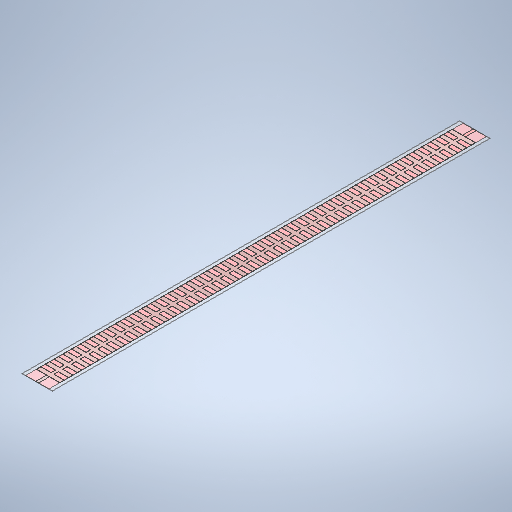
# Autodesk Inventor part: Sensor_completo
Saved by Autodesk Inventor 2025.2 (Build 292293000, 293)
## iProperties
Created: 2025-04-22
Part Number: Sensor_completo
Material: Genérico
Document SubType Name: Modeling
Designer: julia
Density: 1 g/cm^3
Appearance: Transparente - Claro
Author: julia
Autodesk Inventor part; units mm, degrees
ref_plane "YZ Plane" through (0, 0, 0) normal (1, 0, 0) x (0, 1, 0)
ref_plane "XZ Plane" through (0, 0, 0) normal (0, 1, 0) x (-1, 0, 0)
ref_plane "XY Plane" through (0, 0, 0) normal (0, 0, 1) x (1, 0, 0)
sketch "Boceto1" plane through (0, 0, 0) normal (0, 1, 0) x (-1, 0, 0)
  line L0 (0, 0) -> (1.034, 0)
  line L1 (1.026, -15) -> (0, -15)
  line L2 (0, -15) -> (0, 0)
  line L3 (1.034, 0) -> (0.517, 0)
  line L4 (0.517, 0) -> (0.6595, 0)
  line L5 (0.517, 0) -> (0.567, 0)
  line L6 (0.567, 0) -> (0.567, -0.375)
  line L7 (0.567, -0.375) -> (0.917, -0.375)
  line L8 (0.917, -0.375) -> (0.917, -0.525)
  line L9 (0.517, 0) -> (0.467, 0)
  line L10 (0.467, 0) -> (0.467, -0.375)
  line L11 (0.467, -0.375) -> (0.117, -0.375)
  line L12 (0.117, -0.375) -> (0.117, -0.525)
  line L13 (0.117, -0.525) -> (0.467, -0.525)
  line L14 (0.467, -0.525) -> (0.467, -0.675)
  line L15 (0.917, -0.525) -> (0.567, -0.525)
  line L16 (0.567, -0.525) -> (0.567, -0.675)
  line L17 (0.567, -14.625) -> (0.567, -15)
  line L18 (0.467, -14.625) -> (0.467, -15)
  line L19 (0.567, -14.625) -> (0.467, -14.625)
  line L20 (0.567, -0.375) -> (0.467, -0.375)
  line L21 (1.034, -15) -> (1.042, -15)
  line L22 (1.034, -15) -> (1.026, -15)
  line L23 (1.026, -15) -> (1.034, 0)
  line L24 (0.567, -0.675) -> (0.917, -0.675)
  line L25 (0.917, -0.675) -> (0.917, -0.825)
  line L26 (0.917, -0.825) -> (0.567, -0.825)
  line L27 (0.567, -0.825) -> (0.567, -0.975)
  line L28 (0.467, -0.675) -> (0.117, -0.675)
  line L29 (0.117, -0.675) -> (0.117, -0.825)
  line L30 (0.117, -0.825) -> (0.467, -0.825)
  line L31 (0.467, -0.825) -> (0.467, -0.975)
  line L32 (0.567, -0.975) -> (0.917, -0.975)
  line L33 (0.917, -0.975) -> (0.917, -1.125)
  line L34 (0.917, -1.125) -> (0.567, -1.125)
  line L35 (0.567, -1.125) -> (0.567, -1.275)
  line L36 (0.467, -0.975) -> (0.117, -0.975)
  line L37 (0.117, -0.975) -> (0.117, -1.125)
  line L38 (0.117, -1.125) -> (0.467, -1.125)
  line L39 (0.467, -1.125) -> (0.467, -1.275)
  line L40 (0.567, -1.275) -> (0.917, -1.275)
  line L41 (0.917, -1.275) -> (0.917, -1.425)
  line L42 (0.917, -1.425) -> (0.567, -1.425)
  line L43 (0.567, -1.425) -> (0.567, -1.575)
  line L44 (0.467, -1.275) -> (0.117, -1.275)
  line L45 (0.117, -1.275) -> (0.117, -1.425)
  line L46 (0.117, -1.425) -> (0.467, -1.425)
  line L47 (0.467, -1.425) -> (0.467, -1.575)
  line L48 (0.567, -1.575) -> (0.917, -1.575)
  line L49 (0.917, -1.575) -> (0.917, -1.725)
  line L50 (0.917, -1.725) -> (0.567, -1.725)
  line L51 (0.567, -1.725) -> (0.567, -1.875)
  line L52 (0.467, -1.575) -> (0.117, -1.575)
  line L53 (0.117, -1.575) -> (0.117, -1.725)
  line L54 (0.117, -1.725) -> (0.467, -1.725)
  line L55 (0.467, -1.725) -> (0.467, -1.875)
  line L56 (0.567, -1.875) -> (0.917, -1.875)
  line L57 (0.917, -1.875) -> (0.917, -2.025)
  line L58 (0.917, -2.025) -> (0.567, -2.025)
  line L59 (0.567, -2.025) -> (0.567, -2.175)
  line L60 (0.467, -1.875) -> (0.117, -1.875)
  line L61 (0.117, -1.875) -> (0.117, -2.025)
  line L62 (0.117, -2.025) -> (0.467, -2.025)
  line L63 (0.467, -2.025) -> (0.467, -2.175)
  line L64 (0.567, -2.175) -> (0.917, -2.175)
  line L65 (0.917, -2.175) -> (0.917, -2.325)
  line L66 (0.917, -2.325) -> (0.567, -2.325)
  line L67 (0.567, -2.325) -> (0.567, -2.475)
  line L68 (0.467, -2.175) -> (0.117, -2.175)
  line L69 (0.117, -2.175) -> (0.117, -2.325)
  line L70 (0.117, -2.325) -> (0.467, -2.325)
  line L71 (0.467, -2.325) -> (0.467, -2.475)
  line L72 (0.567, -2.475) -> (0.917, -2.475)
  line L73 (0.917, -2.475) -> (0.917, -2.625)
  line L74 (0.917, -2.625) -> (0.567, -2.625)
  line L75 (0.567, -2.625) -> (0.567, -2.775)
  line L76 (0.467, -2.475) -> (0.117, -2.475)
  line L77 (0.117, -2.475) -> (0.117, -2.625)
  line L78 (0.117, -2.625) -> (0.467, -2.625)
  line L79 (0.467, -2.625) -> (0.467, -2.775)
  line L80 (0.567, -2.775) -> (0.917, -2.775)
  line L81 (0.917, -2.775) -> (0.917, -2.925)
  line L82 (0.917, -2.925) -> (0.567, -2.925)
  line L83 (0.567, -2.925) -> (0.567, -3.075)
  line L84 (0.467, -2.775) -> (0.117, -2.775)
  line L85 (0.117, -2.775) -> (0.117, -2.925)
  line L86 (0.117, -2.925) -> (0.467, -2.925)
  line L87 (0.467, -2.925) -> (0.467, -3.075)
  line L88 (0.567, -3.075) -> (0.917, -3.075)
  line L89 (0.917, -3.075) -> (0.917, -3.225)
  line L90 (0.917, -3.225) -> (0.567, -3.225)
  line L91 (0.567, -3.225) -> (0.567, -3.375)
  line L92 (0.467, -3.075) -> (0.117, -3.075)
  line L93 (0.117, -3.075) -> (0.117, -3.225)
  line L94 (0.117, -3.225) -> (0.467, -3.225)
  line L95 (0.467, -3.225) -> (0.467, -3.375)
  line L96 (0.567, -3.375) -> (0.917, -3.375)
  line L97 (0.917, -3.375) -> (0.917, -3.525)
  line L98 (0.917, -3.525) -> (0.567, -3.525)
  line L99 (0.567, -3.525) -> (0.567, -3.675)
  line L100 (0.467, -3.375) -> (0.117, -3.375)
  line L101 (0.117, -3.375) -> (0.117, -3.525)
  line L102 (0.117, -3.525) -> (0.467, -3.525)
  line L103 (0.467, -3.525) -> (0.467, -3.675)
  line L104 (0.567, -3.675) -> (0.917, -3.675)
  line L105 (0.917, -3.675) -> (0.917, -3.825)
  line L106 (0.917, -3.825) -> (0.567, -3.825)
  line L107 (0.567, -3.825) -> (0.567, -3.975)
  line L108 (0.467, -3.675) -> (0.117, -3.675)
  line L109 (0.117, -3.675) -> (0.117, -3.825)
  line L110 (0.117, -3.825) -> (0.467, -3.825)
  line L111 (0.467, -3.825) -> (0.467, -3.975)
  line L112 (0.567, -3.975) -> (0.917, -3.975)
  line L113 (0.917, -3.975) -> (0.917, -4.125)
  line L114 (0.917, -4.125) -> (0.567, -4.125)
  line L115 (0.567, -4.125) -> (0.567, -4.275)
  line L116 (0.467, -3.975) -> (0.117, -3.975)
  line L117 (0.117, -3.975) -> (0.117, -4.125)
  line L118 (0.117, -4.125) -> (0.467, -4.125)
  line L119 (0.467, -4.125) -> (0.467, -4.275)
  line L120 (0.567, -4.275) -> (0.917, -4.275)
  line L121 (0.917, -4.275) -> (0.917, -4.425)
  line L122 (0.917, -4.425) -> (0.567, -4.425)
  line L123 (0.567, -4.425) -> (0.567, -4.575)
  line L124 (0.467, -4.275) -> (0.117, -4.275)
  line L125 (0.117, -4.275) -> (0.117, -4.425)
  line L126 (0.117, -4.425) -> (0.467, -4.425)
  line L127 (0.467, -4.425) -> (0.467, -4.575)
  line L128 (0.567, -4.575) -> (0.917, -4.575)
  line L129 (0.917, -4.575) -> (0.917, -4.725)
  line L130 (0.917, -4.725) -> (0.567, -4.725)
  line L131 (0.567, -4.725) -> (0.567, -4.875)
  line L132 (0.467, -4.575) -> (0.117, -4.575)
  line L133 (0.117, -4.575) -> (0.117, -4.725)
  line L134 (0.117, -4.725) -> (0.467, -4.725)
  line L135 (0.467, -4.725) -> (0.467, -4.875)
  line L136 (0.567, -4.875) -> (0.917, -4.875)
  line L137 (0.917, -4.875) -> (0.917, -5.025)
  line L138 (0.917, -5.025) -> (0.567, -5.025)
  line L139 (0.567, -5.025) -> (0.567, -5.175)
  line L140 (0.467, -4.875) -> (0.117, -4.875)
  line L141 (0.117, -4.875) -> (0.117, -5.025)
  line L142 (0.117, -5.025) -> (0.467, -5.025)
  line L143 (0.467, -5.025) -> (0.467, -5.175)
  line L144 (0.567, -5.175) -> (0.917, -5.175)
  line L145 (0.917, -5.175) -> (0.917, -5.325)
  line L146 (0.917, -5.325) -> (0.567, -5.325)
  line L147 (0.567, -5.325) -> (0.567, -5.475)
  line L148 (0.467, -5.175) -> (0.117, -5.175)
  line L149 (0.117, -5.175) -> (0.117, -5.325)
  line L150 (0.117, -5.325) -> (0.467, -5.325)
  line L151 (0.467, -5.325) -> (0.467, -5.475)
  line L152 (0.567, -5.475) -> (0.917, -5.475)
  line L153 (0.917, -5.475) -> (0.917, -5.625)
  line L154 (0.917, -5.625) -> (0.567, -5.625)
  line L155 (0.567, -5.625) -> (0.567, -5.775)
  line L156 (0.467, -5.475) -> (0.117, -5.475)
  line L157 (0.117, -5.475) -> (0.117, -5.625)
  line L158 (0.117, -5.625) -> (0.467, -5.625)
  line L159 (0.467, -5.625) -> (0.467, -5.775)
  line L160 (0.567, -5.775) -> (0.917, -5.775)
  line L161 (0.917, -5.775) -> (0.917, -5.925)
  line L162 (0.917, -5.925) -> (0.567, -5.925)
  line L163 (0.567, -5.925) -> (0.567, -6.075)
  line L164 (0.467, -5.775) -> (0.117, -5.775)
  line L165 (0.117, -5.775) -> (0.117, -5.925)
  line L166 (0.117, -5.925) -> (0.467, -5.925)
  line L167 (0.467, -5.925) -> (0.467, -6.075)
  line L168 (0.567, -6.075) -> (0.917, -6.075)
  line L169 (0.917, -6.075) -> (0.917, -6.225)
  line L170 (0.917, -6.225) -> (0.567, -6.225)
  line L171 (0.567, -6.225) -> (0.567, -6.375)
  line L172 (0.467, -6.075) -> (0.117, -6.075)
  line L173 (0.117, -6.075) -> (0.117, -6.225)
  line L174 (0.117, -6.225) -> (0.467, -6.225)
  line L175 (0.467, -6.225) -> (0.467, -6.375)
  line L176 (0.567, -6.375) -> (0.917, -6.375)
  line L177 (0.917, -6.375) -> (0.917, -6.525)
  line L178 (0.917, -6.525) -> (0.567, -6.525)
  line L179 (0.567, -6.525) -> (0.567, -6.675)
  line L180 (0.467, -6.375) -> (0.117, -6.375)
  line L181 (0.117, -6.375) -> (0.117, -6.525)
  line L182 (0.117, -6.525) -> (0.467, -6.525)
  line L183 (0.467, -6.525) -> (0.467, -6.675)
  line L184 (0.567, -6.675) -> (0.917, -6.675)
  line L185 (0.917, -6.675) -> (0.917, -6.825)
  line L186 (0.917, -6.825) -> (0.567, -6.825)
  line L187 (0.567, -6.825) -> (0.567, -6.975)
  line L188 (0.467, -6.675) -> (0.117, -6.675)
  line L189 (0.117, -6.675) -> (0.117, -6.825)
  line L190 (0.117, -6.825) -> (0.467, -6.825)
  line L191 (0.467, -6.825) -> (0.467, -6.975)
  line L192 (0.567, -6.975) -> (0.917, -6.975)
  line L193 (0.917, -6.975) -> (0.917, -7.125)
  line L194 (0.917, -7.125) -> (0.567, -7.125)
  line L195 (0.567, -7.125) -> (0.567, -7.275)
  line L196 (0.467, -6.975) -> (0.117, -6.975)
  line L197 (0.117, -6.975) -> (0.117, -7.125)
  line L198 (0.117, -7.125) -> (0.467, -7.125)
  line L199 (0.467, -7.125) -> (0.467, -7.275)
  line L200 (0.567, -7.275) -> (0.917, -7.275)
  line L201 (0.917, -7.275) -> (0.917, -7.425)
  line L202 (0.917, -7.425) -> (0.567, -7.425)
  line L203 (0.567, -7.425) -> (0.567, -7.575)
  line L204 (0.467, -7.275) -> (0.117, -7.275)
  line L205 (0.117, -7.275) -> (0.117, -7.425)
  line L206 (0.117, -7.425) -> (0.467, -7.425)
  line L207 (0.467, -7.425) -> (0.467, -7.575)
  line L208 (0.567, -7.575) -> (0.917, -7.575)
  line L209 (0.917, -7.575) -> (0.917, -7.725)
  line L210 (0.917, -7.725) -> (0.567, -7.725)
  line L211 (0.567, -7.725) -> (0.567, -7.875)
  line L212 (0.467, -7.575) -> (0.117, -7.575)
  line L213 (0.117, -7.575) -> (0.117, -7.725)
  line L214 (0.117, -7.725) -> (0.467, -7.725)
  line L215 (0.467, -7.725) -> (0.467, -7.875)
  line L216 (0.567, -7.875) -> (0.917, -7.875)
  line L217 (0.917, -7.875) -> (0.917, -8.025)
  line L218 (0.917, -8.025) -> (0.567, -8.025)
  line L219 (0.567, -8.025) -> (0.567, -8.175)
  line L220 (0.467, -7.875) -> (0.117, -7.875)
  line L221 (0.117, -7.875) -> (0.117, -8.025)
  line L222 (0.117, -8.025) -> (0.467, -8.025)
  line L223 (0.467, -8.025) -> (0.467, -8.175)
  line L224 (0.567, -8.175) -> (0.917, -8.175)
  line L225 (0.917, -8.175) -> (0.917, -8.325)
  line L226 (0.917, -8.325) -> (0.567, -8.325)
  line L227 (0.567, -8.325) -> (0.567, -8.475)
  line L228 (0.467, -8.175) -> (0.117, -8.175)
  line L229 (0.117, -8.175) -> (0.117, -8.325)
  line L230 (0.117, -8.325) -> (0.467, -8.325)
  line L231 (0.467, -8.325) -> (0.467, -8.475)
  line L232 (0.567, -8.475) -> (0.917, -8.475)
  line L233 (0.917, -8.475) -> (0.917, -8.625)
  line L234 (0.917, -8.625) -> (0.567, -8.625)
  line L235 (0.567, -8.625) -> (0.567, -8.775)
  line L236 (0.467, -8.475) -> (0.117, -8.475)
  line L237 (0.117, -8.475) -> (0.117, -8.625)
  line L238 (0.117, -8.625) -> (0.467, -8.625)
  line L239 (0.467, -8.625) -> (0.467, -8.775)
  line L240 (0.567, -8.775) -> (0.917, -8.775)
  line L241 (0.917, -8.775) -> (0.917, -8.925)
  line L242 (0.917, -8.925) -> (0.567, -8.925)
  line L243 (0.567, -8.925) -> (0.567, -9.075)
  line L244 (0.467, -8.775) -> (0.117, -8.775)
  line L245 (0.117, -8.775) -> (0.117, -8.925)
  line L246 (0.117, -8.925) -> (0.467, -8.925)
  line L247 (0.467, -8.925) -> (0.467, -9.075)
  line L248 (0.567, -9.075) -> (0.917, -9.075)
  line L249 (0.917, -9.075) -> (0.917, -9.225)
  line L250 (0.917, -9.225) -> (0.567, -9.225)
  line L251 (0.567, -9.225) -> (0.567, -9.375)
  line L252 (0.467, -9.075) -> (0.117, -9.075)
  line L253 (0.117, -9.075) -> (0.117, -9.225)
  line L254 (0.117, -9.225) -> (0.467, -9.225)
  line L255 (0.467, -9.225) -> (0.467, -9.375)
  line L256 (0.567, -9.375) -> (0.917, -9.375)
  line L257 (0.917, -9.375) -> (0.917, -9.525)
  line L258 (0.917, -9.525) -> (0.567, -9.525)
  line L259 (0.567, -9.525) -> (0.567, -9.675)
  line L260 (0.467, -9.375) -> (0.117, -9.375)
  line L261 (0.117, -9.375) -> (0.117, -9.525)
  line L262 (0.117, -9.525) -> (0.467, -9.525)
  line L263 (0.467, -9.525) -> (0.467, -9.675)
  line L264 (0.567, -9.675) -> (0.917, -9.675)
  line L265 (0.917, -9.675) -> (0.917, -9.825)
  line L266 (0.917, -9.825) -> (0.567, -9.825)
  line L267 (0.567, -9.825) -> (0.567, -9.975)
  line L268 (0.467, -9.675) -> (0.117, -9.675)
  line L269 (0.117, -9.675) -> (0.117, -9.825)
  line L270 (0.117, -9.825) -> (0.467, -9.825)
  line L271 (0.467, -9.825) -> (0.467, -9.975)
  line L272 (0.567, -9.975) -> (0.917, -9.975)
  line L273 (0.917, -9.975) -> (0.917, -10.125)
  line L274 (0.917, -10.125) -> (0.567, -10.125)
  line L275 (0.567, -10.125) -> (0.567, -10.275)
  line L276 (0.467, -9.975) -> (0.117, -9.975)
  line L277 (0.117, -9.975) -> (0.117, -10.125)
  line L278 (0.117, -10.125) -> (0.467, -10.125)
  line L279 (0.467, -10.125) -> (0.467, -10.275)
  line L280 (0.567, -10.275) -> (0.917, -10.275)
  line L281 (0.917, -10.275) -> (0.917, -10.425)
  line L282 (0.917, -10.425) -> (0.567, -10.425)
  line L283 (0.567, -10.425) -> (0.567, -10.575)
  line L284 (0.467, -10.275) -> (0.117, -10.275)
  line L285 (0.117, -10.275) -> (0.117, -10.425)
  line L286 (0.117, -10.425) -> (0.467, -10.425)
  line L287 (0.467, -10.425) -> (0.467, -10.575)
  line L288 (0.567, -10.575) -> (0.917, -10.575)
  line L289 (0.917, -10.575) -> (0.917, -10.725)
  line L290 (0.917, -10.725) -> (0.567, -10.725)
  line L291 (0.567, -10.725) -> (0.567, -10.875)
  line L292 (0.467, -10.575) -> (0.117, -10.575)
  line L293 (0.117, -10.575) -> (0.117, -10.725)
  line L294 (0.117, -10.725) -> (0.467, -10.725)
  line L295 (0.467, -10.725) -> (0.467, -10.875)
  line L296 (0.567, -10.875) -> (0.917, -10.875)
  line L297 (0.917, -10.875) -> (0.917, -11.025)
  line L298 (0.917, -11.025) -> (0.567, -11.025)
  line L299 (0.567, -11.025) -> (0.567, -11.175)
  line L300 (0.467, -10.875) -> (0.117, -10.875)
  line L301 (0.117, -10.875) -> (0.117, -11.025)
  line L302 (0.117, -11.025) -> (0.467, -11.025)
  line L303 (0.467, -11.025) -> (0.467, -11.175)
  line L304 (0.567, -11.175) -> (0.917, -11.175)
  line L305 (0.917, -11.175) -> (0.917, -11.325)
  line L306 (0.917, -11.325) -> (0.567, -11.325)
  line L307 (0.567, -11.325) -> (0.567, -11.475)
  line L308 (0.467, -11.175) -> (0.117, -11.175)
  line L309 (0.117, -11.175) -> (0.117, -11.325)
  line L310 (0.117, -11.325) -> (0.467, -11.325)
  line L311 (0.467, -11.325) -> (0.467, -11.475)
  line L312 (0.567, -11.475) -> (0.917, -11.475)
  line L313 (0.917, -11.475) -> (0.917, -11.625)
  line L314 (0.917, -11.625) -> (0.567, -11.625)
  line L315 (0.567, -11.625) -> (0.567, -11.775)
  line L316 (0.467, -11.475) -> (0.117, -11.475)
  line L317 (0.117, -11.475) -> (0.117, -11.625)
  line L318 (0.117, -11.625) -> (0.467, -11.625)
  line L319 (0.467, -11.625) -> (0.467, -11.775)
  line L320 (0.567, -11.775) -> (0.917, -11.775)
  line L321 (0.917, -11.775) -> (0.917, -11.925)
  line L322 (0.917, -11.925) -> (0.567, -11.925)
  line L323 (0.567, -11.925) -> (0.567, -12.075)
  line L324 (0.467, -11.775) -> (0.117, -11.775)
  line L325 (0.117, -11.775) -> (0.117, -11.925)
  line L326 (0.117, -11.925) -> (0.467, -11.925)
  line L327 (0.467, -11.925) -> (0.467, -12.075)
  line L328 (0.567, -12.075) -> (0.917, -12.075)
  line L329 (0.917, -12.075) -> (0.917, -12.225)
  line L330 (0.917, -12.225) -> (0.567, -12.225)
  line L331 (0.567, -12.225) -> (0.567, -12.375)
  line L332 (0.467, -12.075) -> (0.117, -12.075)
  line L333 (0.117, -12.075) -> (0.117, -12.225)
  line L334 (0.117, -12.225) -> (0.467, -12.225)
  line L335 (0.467, -12.225) -> (0.467, -12.375)
  line L336 (0.567, -12.375) -> (0.917, -12.375)
  line L337 (0.917, -12.375) -> (0.917, -12.525)
  line L338 (0.917, -12.525) -> (0.567, -12.525)
  line L339 (0.567, -12.525) -> (0.567, -12.675)
  line L340 (0.467, -12.375) -> (0.117, -12.375)
  line L341 (0.117, -12.375) -> (0.117, -12.525)
  line L342 (0.117, -12.525) -> (0.467, -12.525)
  line L343 (0.467, -12.525) -> (0.467, -12.675)
  line L344 (0.567, -12.675) -> (0.917, -12.675)
  line L345 (0.917, -12.675) -> (0.917, -12.825)
  line L346 (0.917, -12.825) -> (0.567, -12.825)
  line L347 (0.567, -12.825) -> (0.567, -12.975)
  line L348 (0.467, -12.675) -> (0.117, -12.675)
  line L349 (0.117, -12.675) -> (0.117, -12.825)
  line L350 (0.117, -12.825) -> (0.467, -12.825)
  line L351 (0.467, -12.825) -> (0.467, -12.975)
  line L352 (0.567, -12.975) -> (0.917, -12.975)
  line L353 (0.917, -12.975) -> (0.917, -13.125)
  line L354 (0.917, -13.125) -> (0.567, -13.125)
  line L355 (0.567, -13.125) -> (0.567, -13.275)
  line L356 (0.467, -12.975) -> (0.117, -12.975)
  line L357 (0.117, -12.975) -> (0.117, -13.125)
  line L358 (0.117, -13.125) -> (0.467, -13.125)
  line L359 (0.467, -13.125) -> (0.467, -13.275)
  line L360 (0.567, -13.275) -> (0.917, -13.275)
  line L361 (0.917, -13.275) -> (0.917, -13.425)
  line L362 (0.917, -13.425) -> (0.567, -13.425)
  line L363 (0.567, -13.425) -> (0.567, -13.575)
  line L364 (0.467, -13.275) -> (0.117, -13.275)
  line L365 (0.117, -13.275) -> (0.117, -13.425)
  line L366 (0.117, -13.425) -> (0.467, -13.425)
  line L367 (0.467, -13.425) -> (0.467, -13.575)
  line L368 (0.567, -13.575) -> (0.917, -13.575)
  line L369 (0.917, -13.575) -> (0.917, -13.725)
  line L370 (0.917, -13.725) -> (0.567, -13.725)
  line L371 (0.567, -13.725) -> (0.567, -13.875)
  line L372 (0.467, -13.575) -> (0.117, -13.575)
  line L373 (0.117, -13.575) -> (0.117, -13.725)
  line L374 (0.117, -13.725) -> (0.467, -13.725)
  line L375 (0.467, -13.725) -> (0.467, -13.875)
  line L376 (0.567, -13.875) -> (0.917, -13.875)
  line L377 (0.917, -13.875) -> (0.917, -14.025)
  line L378 (0.917, -14.025) -> (0.567, -14.025)
  line L379 (0.567, -14.025) -> (0.567, -14.175)
  line L380 (0.467, -13.875) -> (0.117, -13.875)
  line L381 (0.117, -13.875) -> (0.117, -14.025)
  line L382 (0.117, -14.025) -> (0.467, -14.025)
  line L383 (0.467, -14.025) -> (0.467, -14.175)
  line L384 (0.567, -14.175) -> (0.917, -14.175)
  line L385 (0.917, -14.175) -> (0.917, -14.325)
  line L386 (0.917, -14.325) -> (0.567, -14.325)
  line L387 (0.567, -14.325) -> (0.567, -14.475)
  line L388 (0.467, -14.175) -> (0.117, -14.175)
  line L389 (0.117, -14.175) -> (0.117, -14.325)
  line L390 (0.117, -14.325) -> (0.467, -14.325)
  line L391 (0.467, -14.325) -> (0.467, -14.475)
  line L392 (0.567, -14.475) -> (0.917, -14.475)
  line L393 (0.917, -14.475) -> (0.917, -14.625)
  line L394 (0.917, -14.625) -> (0.567, -14.625)
  line L395 (0.567, -14.625) -> (0.567, -14.775)
  line L396 (0.467, -14.475) -> (0.117, -14.475)
  line L397 (0.117, -14.475) -> (0.117, -14.625)
  line L398 (0.117, -14.625) -> (0.467, -14.625)
  line L399 (0.467, -14.625) -> (0.467, -14.775)
  line L400 (0.117, -0.375) -> (0.917, -0.375)
  line L401 (0.917, -0.375) -> (0.917, -15)
  line L402 (0.917, -15) -> (0.117, -15)
  line L403 (0.117, -15) -> (0.117, -0.375)
  line L404 (0.117, 0) -> (0.917, 0)
  line L405 (0.917, 0) -> (0.917, -14.625)
  line L406 (0.917, -14.625) -> (0.117, -14.625)
  line L407 (0.117, -14.625) -> (0.117, 0)
  point P0 (0.117, -0.675)
  point P1 (0.117, -0.975)
  point P2 (0.117, -1.575)
  point P3 (0.117, -1.875)
  point P4 (0.117, -2.475)
  point P5 (0.117, -2.775)
  point P6 (0.117, -3.375)
  point P7 (0.117, -3.675)
  point P8 (0.117, -4.275)
  point P9 (0.117, -4.575)
  point P10 (0.117, -4.875)
  point P11 (0.117, -5.175)
  point P12 (0.117, -5.475)
  point P13 (0.117, -5.775)
  point P14 (0.117, -6.075)
  point P15 (0.117, -6.375)
  point P16 (0.117, -6.675)
  point P17 (0.117, -7.275)
  point P18 (0.117, -7.575)
  point P19 (0.117, -8.175)
  point P20 (0.117, -8.475)
  point P21 (0.117, -9.075)
  point P22 (0.117, -9.375)
  point P23 (0.117, -9.975)
  point P24 (0.117, -10.275)
  point P25 (0.117, -10.875)
  point P26 (0.117, -11.175)
  point P27 (0.117, -11.775)
  point P28 (0.117, -12.075)
  point P29 (0.117, -12.675)
  point P30 (0.117, -12.975)
  point P31 (0.117, -13.575)
  point P32 (0.117, -13.875)
  point P33 (0.117, -14.475)
  dimension "d0" = 1.034
  dimension "d1" = 15
  dimension "d2" = 0.517
  dimension "d3" = 0.05
  dimension "d4" = 0.375
  dimension "d5" = 0.35
  dimension "d6" = 0.15
  dimension "d7" = 0.05
  dimension "d8" = 0.35
  dimension "d9" = 0.15
  dimension "d10" = 0.15
  dimension "d18" = 0.375
  dimension "d19" = 0.375
  dimension "d24" = 0.3
  constraints: 812 end point, 10 perpendicular, 9 point on line, 5 horizontal, 3 vertical, 2 collinear, 1 midpoint, 1 parallel, 849 other
  measures "d0" distance of L0.start L0.end
  measures "d1" distance of L0.end L21.start
  measures "d2" distance of L0.end L3.end
  measures "d3" distance of L3.end L5.end
  measures "d4" distance of L5.end L6.end
  measures "d5" distance of L6.end L7.end
  measures "d6" distance of L7.end L8.end
  measures "d7" distance of L3.end L9.end
  measures "d8" distance of L10.end L11.end
  measures "d9" distance of L11.end L12.end
  measures "d10" distance of L13.end L14.end
  measures "d18" distance of L9.end L10.end
  measures "d19" distance of L17.end L17.start
  measures "d24" distance of L6.end L24.start
extrude "Extrusión4" add sketch "Boceto1" along normal blind 0.0025 contours L11 L20 L7 L8 L15 L16 L24 L25 L26 L27 L32 L33 L34 L35 L40 L41 L42 L43 L48 L49 L50 L51 L56 L57 L58 L59 L64 L65 L66 L67 L72 L73 L74 L75 L80 L81 L82 L83 L88 L89 L90 L91 L96 L97 L98 L99 L104 L105 L106 L107 L112 L113 L114 L115 L120 L121 L122 L123 L128 L129 L130 L131 L136 L137 L138 L139 L144 L145 L146 L147 L152 L153 L154 L155 L160 L161 L162 L163 L168 L169 L170 L171 L176 L177 L178 L179 L184 L185 L186 L187 L192 L193 L194 L195 L200 L201 L202 L203 L208 L209 L210 L211 L216 L217 L218 L219 L224 L225 L226 L227 L232 L233 L234 L235 L240 L241 L242 L243 L248 L249 L250 L251 L256 L257 L258 L259 L264 L265 L266 L267 L272 L273 L274 L275 L280 L281 L282 L283 L288 L289 L290 L291 L296 L297 L298 L299 L304 L305 L306 L307 L312 L313 L314 L315 L320 L321 L322 L323 L328 L329 L330 L331 L336 L337 L338 L339 L344 L345 L346 L347 L352 L353 L354 L355 L360 L361 L362 L363 L368 L369 L370 L371 L376 L377 L378 L379 L384 L385 L386 L387 L392 L393 L394 L19 L398 L397 L396 L391 L390 L389 L388 L383 L382 L381 L380 L375 L374 L373 L372 L367 L366 L365 L364 L359 L358 L357 L356 L351 L350 L349 L348 L343 L342 L341 L340 L335 L334 L333 L332 L327 L326 L325 L324 L319 L318 L317 L316 L311 L310 L309 L308 L303 L302 L301 L300 L295 L294 L293 L292 L287 L286 L285 L284 L279 L278 L277 L276 L271 L270 L269 L268 L263 L262 L261 L260 L255 L254 L253 L252 L247 L246 L245 L244 L239 L238 L237 L236 L231 L230 L229 L228 L223 L222 L221 L220 L215 L214 L213 L212 L207 L206 L205 L204 L199 L198 L197 L196 L191 L190 L189 L188 L183 L182 L181 L180 L175 L174 L173 L172 L167 L166 L165 L164 L159 L158 L157 L156 L151 L150 L149 L148 L143 L142 L141 L140 L135 L134 L133 L132 L127 L126 L125 L124 L119 L118 L117 L116 L111 L110 L109 L108 L103 L102 L101 L100 L95 L94 L93 L92 L87 L86 L85 L84 L79 L78 L77 L76 L71 L70 L69 L68 L63 L62 L61 L60 L55 L54 L53 L52 L47 L46 L45 L44 L39 L38 L37 L36 L31 L30 L29 L28 L14 L13 L12 | L403 L398 L18 L1 | L13 L14 L28 L403 | L18 L19 L17 L1 | L17 L394 L401 L1 | L403 L390 L391 L396 | L30 L31 L36 L403 | L401 L24 L16 L15 | L403 L382 L383 L388 | L38 L39 L44 L403 | L392 L387 L386 L401 | L401 L32 L27 L26 | L403 L374 L375 L380 | L46 L47 L52 L403 | L384 L379 L378 L401 | L401 L40 L35 L34 | L403 L366 L367 L372 | L54 L55 L60 L403 | L376 L371 L370 L401 | L401 L48 L43 L42 | L403 L358 L359 L364 | L62 L63 L68 L403 | L368 L363 L362 L401 | L401 L56 L51 L50 | L403 L350 L351 L356 | L70 L71 L76 L403 | L360 L355 L354 L401 | L401 L64 L59 L58 | L403 L342 L343 L348 | L78 L79 L84 L403 | L352 L347 L346 L401 | L401 L72 L67 L66 | L403 L334 L335 L340 | L86 L87 L92 L403 | L344 L339 L338 L401 | L401 L80 L75 L74 | L403 L326 L327 L332 | L94 L95 L100 L403 | L336 L331 L330 L401 | L401 L88 L83 L82 | L403 L318 L319 L324 | L102 L103 L108 L403 | L328 L323 L322 L401 | L401 L96 L91 L90 | L403 L310 L311 L316 | L110 L111 L116 L403 | L320 L315 L314 L401 | L401 L104 L99 L98 | L403 L302 L303 L308 | L118 L119 L124 L403 | L312 L307 L306 L401 | L401 L112 L107 L106 | L403 L294 L295 L300 | L126 L127 L132 L403 | L304 L299 L298 L401 | L401 L120 L115 L114 | L403 L286 L287 L292 | L134 L135 L140 L403 | L296 L291 L290 L401 | L401 L128 L123 L122 | L403 L278 L279 L284 | L142 L143 L148 L403 | L288 L283 L282 L401 | L401 L136 L131 L130 | L403 L270 L271 L276 | L150 L151 L156 L403 | L280 L275 L274 L401 | L401 L144 L139 L138 | L403 L262 L263 L268 | L158 L159 L164 L403 | L272 L267 L266 L401 | L401 L152 L147 L146 | L403 L254 L255 L260 | L166 L167 L172 L403 | L264 L259 L258 L401 | L401 L160 L155 L154 | L403 L246 L247 L252 | L174 L175 L180 L403 | L256 L251 L250 L401 | L401 L168 L163 L162 | L403 L238 L239 L244 | L182 L183 L188 L403 | L248 L243 L242 L401 | L401 L176 L171 L170 | L403 L230 L231 L236 | L190 L191 L196 L403 | L240 L235 L234 L401 | L401 L184 L179 L178 | L403 L222 L223 L228 | L198 L199 L204 L403 | L232 L227 L226 L401 | L401 L192 L187 L186 | L403 L214 L215 L220 | L206 L207 L212 L403 | L224 L219 L218 L401 | L401 L200 L195 L194 | L216 L211 L210 L401 | L401 L208 L203 L202
extrude "Extrusión5" add sketch "Boceto1" along normal blind 0.001 from surface at 0.0025 separate body contours L11 L20 L7 L8 L15 L16 L24 L25 L26 L27 L32 L33 L34 L35 L40 L41 L42 L43 L48 L49 L50 L51 L56 L57 L58 L59 L64 L65 L66 L67 L72 L73 L74 L75 L80 L81 L82 L83 L88 L89 L90 L91 L96 L97 L98 L99 L104 L105 L106 L107 L112 L113 L114 L115 L120 L121 L122 L123 L128 L129 L130 L131 L136 L137 L138 L139 L144 L145 L146 L147 L152 L153 L154 L155 L160 L161 L162 L163 L168 L169 L170 L171 L176 L177 L178 L179 L184 L185 L186 L187 L192 L193 L194 L195 L200 L201 L202 L203 L208 L209 L210 L211 L216 L217 L218 L219 L224 L225 L226 L227 L232 L233 L234 L235 L240 L241 L242 L243 L248 L249 L250 L251 L256 L257 L258 L259 L264 L265 L266 L267 L272 L273 L274 L275 L280 L281 L282 L283 L288 L289 L290 L291 L296 L297 L298 L299 L304 L305 L306 L307 L312 L313 L314 L315 L320 L321 L322 L323 L328 L329 L330 L331 L336 L337 L338 L339 L344 L345 L346 L347 L352 L353 L354 L355 L360 L361 L362 L363 L368 L369 L370 L371 L376 L377 L378 L379 L384 L385 L386 L387 L392 L393 L394 L19 L398 L397 L396 L391 L390 L389 L388 L383 L382 L381 L380 L375 L374 L373 L372 L367 L366 L365 L364 L359 L358 L357 L356 L351 L350 L349 L348 L343 L342 L341 L340 L335 L334 L333 L332 L327 L326 L325 L324 L319 L318 L317 L316 L311 L310 L309 L308 L303 L302 L301 L300 L295 L294 L293 L292 L287 L286 L285 L284 L279 L278 L277 L276 L271 L270 L269 L268 L263 L262 L261 L260 L255 L254 L253 L252 L247 L246 L245 L244 L239 L238 L237 L236 L231 L230 L229 L228 L223 L222 L221 L220 L215 L214 L213 L212 L207 L206 L205 L204 L199 L198 L197 L196 L191 L190 L189 L188 L183 L182 L181 L180 L175 L174 L173 L172 L167 L166 L165 L164 L159 L158 L157 L156 L151 L150 L149 L148 L143 L142 L141 L140 L135 L134 L133 L132 L127 L126 L125 L124 L119 L118 L117 L116 L111 L110 L109 L108 L103 L102 L101 L100 L95 L94 L93 L92 L87 L86 L85 L84 L79 L78 L77 L76 L71 L70 L69 L68 L63 L62 L61 L60 L55 L54 L53 L52 L47 L46 L45 L44 L39 L38 L37 L36 L31 L30 L29 L28 L14 L13 L12 | L18 L19 L17 L1
extrude "Extrusión6" add sketch "Boceto1" along normal blind 0.0025 from surface at 0.0035 separate body contours L11 L20 L7 L8 L15 L16 L24 L25 L26 L27 L32 L33 L34 L35 L40 L41 L42 L43 L48 L49 L50 L51 L56 L57 L58 L59 L64 L65 L66 L67 L72 L73 L74 L75 L80 L81 L82 L83 L88 L89 L90 L91 L96 L97 L98 L99 L104 L105 L106 L107 L112 L113 L114 L115 L120 L121 L122 L123 L128 L129 L130 L131 L136 L137 L138 L139 L144 L145 L146 L147 L152 L153 L154 L155 L160 L161 L162 L163 L168 L169 L170 L171 L176 L177 L178 L179 L184 L185 L186 L187 L192 L193 L194 L195 L200 L201 L202 L203 L208 L209 L210 L211 L216 L217 L218 L219 L224 L225 L226 L227 L232 L233 L234 L235 L240 L241 L242 L243 L248 L249 L250 L251 L256 L257 L258 L259 L264 L265 L266 L267 L272 L273 L274 L275 L280 L281 L282 L283 L288 L289 L290 L291 L296 L297 L298 L299 L304 L305 L306 L307 L312 L313 L314 L315 L320 L321 L322 L323 L328 L329 L330 L331 L336 L337 L338 L339 L344 L345 L346 L347 L352 L353 L354 L355 L360 L361 L362 L363 L368 L369 L370 L371 L376 L377 L378 L379 L384 L385 L386 L387 L392 L393 L394 L19 L398 L397 L396 L391 L390 L389 L388 L383 L382 L381 L380 L375 L374 L373 L372 L367 L366 L365 L364 L359 L358 L357 L356 L351 L350 L349 L348 L343 L342 L341 L340 L335 L334 L333 L332 L327 L326 L325 L324 L319 L318 L317 L316 L311 L310 L309 L308 L303 L302 L301 L300 L295 L294 L293 L292 L287 L286 L285 L284 L279 L278 L277 L276 L271 L270 L269 L268 L263 L262 L261 L260 L255 L254 L253 L252 L247 L246 L245 L244 L239 L238 L237 L236 L231 L230 L229 L228 L223 L222 L221 L220 L215 L214 L213 L212 L207 L206 L205 L204 L199 L198 L197 L196 L191 L190 L189 L188 L183 L182 L181 L180 L175 L174 L173 L172 L167 L166 L165 L164 L159 L158 L157 L156 L151 L150 L149 L148 L143 L142 L141 L140 L135 L134 L133 L132 L127 L126 L125 L124 L119 L118 L117 L116 L111 L110 L109 L108 L103 L102 L101 L100 L95 L94 L93 L92 L87 L86 L85 L84 L79 L78 L77 L76 L71 L70 L69 L68 L63 L62 L61 L60 L55 L54 L53 L52 L47 L46 L45 L44 L39 L38 L37 L36 L31 L30 L29 L28 L14 L13 L12 | L18 L19 L17 L1
extrude "Extrusión7" add sketch "Boceto1" along normal blind 0.0025 from surface at 0.006 separate body contours L0 L10 L11 L407 | L0 L6 L20 L10 | L11 L20 L7 L8 L15 L16 L24 L25 L26 L27 L32 L33 L34 L35 L40 L41 L42 L43 L48 L49 L50 L51 L56 L57 L58 L59 L64 L65 L66 L67 L72 L73 L74 L75 L80 L81 L82 L83 L88 L89 L90 L91 L96 L97 L98 L99 L104 L105 L106 L107 L112 L113 L114 L115 L120 L121 L122 L123 L128 L129 L130 L131 L136 L137 L138 L139 L144 L145 L146 L147 L152 L153 L154 L155 L160 L161 L162 L163 L168 L169 L170 L171 L176 L177 L178 L179 L184 L185 L186 L187 L192 L193 L194 L195 L200 L201 L202 L203 L208 L209 L210 L211 L216 L217 L218 L219 L224 L225 L226 L227 L232 L233 L234 L235 L240 L241 L242 L243 L248 L249 L250 L251 L256 L257 L258 L259 L264 L265 L266 L267 L272 L273 L274 L275 L280 L281 L282 L283 L288 L289 L290 L291 L296 L297 L298 L299 L304 L305 L306 L307 L312 L313 L314 L315 L320 L321 L322 L323 L328 L329 L330 L331 L336 L337 L338 L339 L344 L345 L346 L347 L352 L353 L354 L355 L360 L361 L362 L363 L368 L369 L370 L371 L376 L377 L378 L379 L384 L385 L386 L387 L392 L393 L394 L19 L398 L397 L396 L391 L390 L389 L388 L383 L382 L381 L380 L375 L374 L373 L372 L367 L366 L365 L364 L359 L358 L357 L356 L351 L350 L349 L348 L343 L342 L341 L340 L335 L334 L333 L332 L327 L326 L325 L324 L319 L318 L317 L316 L311 L310 L309 L308 L303 L302 L301 L300 L295 L294 L293 L292 L287 L286 L285 L284 L279 L278 L277 L276 L271 L270 L269 L268 L263 L262 L261 L260 L255 L254 L253 L252 L247 L246 L245 L244 L239 L238 L237 L236 L231 L230 L229 L228 L223 L222 L221 L220 L215 L214 L213 L212 L207 L206 L205 L204 L199 L198 L197 L196 L191 L190 L189 L188 L183 L182 L181 L180 L175 L174 L173 L172 L167 L166 L165 L164 L159 L158 L157 L156 L151 L150 L149 L148 L143 L142 L141 L140 L135 L134 L133 L132 L127 L126 L125 L124 L119 L118 L117 L116 L111 L110 L109 L108 L103 L102 L101 L100 L95 L94 L93 L92 L87 L86 L85 L84 L79 L78 L77 L76 L71 L70 L69 L68 L63 L62 L61 L60 L55 L54 L53 L52 L47 L46 L45 L44 L39 L38 L37 L36 L31 L30 L29 L28 L14 L13 L12 | L13 L14 L28 L403 | L0 L405 L7 L6 | L403 L390 L391 L396 | L30 L31 L36 L403 | L401 L24 L16 L15 | L403 L382 L383 L388 | L38 L39 L44 L403 | L392 L387 L386 L401 | L401 L32 L27 L26 | L403 L374 L375 L380 | L46 L47 L52 L403 | L384 L379 L378 L401 | L401 L40 L35 L34 | L403 L366 L367 L372 | L54 L55 L60 L403 | L376 L371 L370 L401 | L401 L48 L43 L42 | L403 L358 L359 L364 | L62 L63 L68 L403 | L368 L363 L362 L401 | L401 L56 L51 L50 | L403 L350 L351 L356 | L70 L71 L76 L403 | L360 L355 L354 L401 | L401 L64 L59 L58 | L403 L342 L343 L348 | L78 L79 L84 L403 | L352 L347 L346 L401 | L401 L72 L67 L66 | L403 L334 L335 L340 | L86 L87 L92 L403 | L344 L339 L338 L401 | L401 L80 L75 L74 | L403 L326 L327 L332 | L94 L95 L100 L403 | L336 L331 L330 L401 | L401 L88 L83 L82 | L403 L318 L319 L324 | L102 L103 L108 L403 | L328 L323 L322 L401 | L401 L96 L91 L90 | L403 L310 L311 L316 | L110 L111 L116 L403 | L320 L315 L314 L401 | L401 L104 L99 L98 | L403 L302 L303 L308 | L118 L119 L124 L403 | L312 L307 L306 L401 | L401 L112 L107 L106 | L403 L294 L295 L300 | L126 L127 L132 L403 | L304 L299 L298 L401 | L401 L120 L115 L114 | L403 L286 L287 L292 | L134 L135 L140 L403 | L296 L291 L290 L401 | L401 L128 L123 L122 | L403 L278 L279 L284 | L142 L143 L148 L403 | L288 L283 L282 L401 | L401 L136 L131 L130 | L403 L270 L271 L276 | L150 L151 L156 L403 | L280 L275 L274 L401 | L401 L144 L139 L138 | L403 L262 L263 L268 | L158 L159 L164 L403 | L272 L267 L266 L401 | L401 L152 L147 L146 | L403 L254 L255 L260 | L166 L167 L172 L403 | L264 L259 L258 L401 | L401 L160 L155 L154 | L403 L246 L247 L252 | L174 L175 L180 L403 | L256 L251 L250 L401 | L401 L168 L163 L162 | L403 L238 L239 L244 | L182 L183 L188 L403 | L248 L243 L242 L401 | L401 L176 L171 L170 | L403 L230 L231 L236 | L190 L191 L196 L403 | L240 L235 L234 L401 | L401 L184 L179 L178 | L403 L222 L223 L228 | L198 L199 L204 L403 | L232 L227 L226 L401 | L401 L192 L187 L186 | L403 L214 L215 L220 | L206 L207 L212 L403 | L224 L219 L218 L401 | L401 L200 L195 L194 | L216 L211 L210 L401 | L401 L208 L203 L202
extrude "Extrusión8" add sketch "Boceto1" along normal blind 0.001 from surface at 0.0085 separate body contours L0 L6 L20 L10 | L11 L20 L7 L8 L15 L16 L24 L25 L26 L27 L32 L33 L34 L35 L40 L41 L42 L43 L48 L49 L50 L51 L56 L57 L58 L59 L64 L65 L66 L67 L72 L73 L74 L75 L80 L81 L82 L83 L88 L89 L90 L91 L96 L97 L98 L99 L104 L105 L106 L107 L112 L113 L114 L115 L120 L121 L122 L123 L128 L129 L130 L131 L136 L137 L138 L139 L144 L145 L146 L147 L152 L153 L154 L155 L160 L161 L162 L163 L168 L169 L170 L171 L176 L177 L178 L179 L184 L185 L186 L187 L192 L193 L194 L195 L200 L201 L202 L203 L208 L209 L210 L211 L216 L217 L218 L219 L224 L225 L226 L227 L232 L233 L234 L235 L240 L241 L242 L243 L248 L249 L250 L251 L256 L257 L258 L259 L264 L265 L266 L267 L272 L273 L274 L275 L280 L281 L282 L283 L288 L289 L290 L291 L296 L297 L298 L299 L304 L305 L306 L307 L312 L313 L314 L315 L320 L321 L322 L323 L328 L329 L330 L331 L336 L337 L338 L339 L344 L345 L346 L347 L352 L353 L354 L355 L360 L361 L362 L363 L368 L369 L370 L371 L376 L377 L378 L379 L384 L385 L386 L387 L392 L393 L394 L19 L398 L397 L396 L391 L390 L389 L388 L383 L382 L381 L380 L375 L374 L373 L372 L367 L366 L365 L364 L359 L358 L357 L356 L351 L350 L349 L348 L343 L342 L341 L340 L335 L334 L333 L332 L327 L326 L325 L324 L319 L318 L317 L316 L311 L310 L309 L308 L303 L302 L301 L300 L295 L294 L293 L292 L287 L286 L285 L284 L279 L278 L277 L276 L271 L270 L269 L268 L263 L262 L261 L260 L255 L254 L253 L252 L247 L246 L245 L244 L239 L238 L237 L236 L231 L230 L229 L228 L223 L222 L221 L220 L215 L214 L213 L212 L207 L206 L205 L204 L199 L198 L197 L196 L191 L190 L189 L188 L183 L182 L181 L180 L175 L174 L173 L172 L167 L166 L165 L164 L159 L158 L157 L156 L151 L150 L149 L148 L143 L142 L141 L140 L135 L134 L133 L132 L127 L126 L125 L124 L119 L118 L117 L116 L111 L110 L109 L108 L103 L102 L101 L100 L95 L94 L93 L92 L87 L86 L85 L84 L79 L78 L77 L76 L71 L70 L69 L68 L63 L62 L61 L60 L55 L54 L53 L52 L47 L46 L45 L44 L39 L38 L37 L36 L31 L30 L29 L28 L14 L13 L12
extrude "Extrusión9" add sketch "Boceto1" along normal blind 0.0025 from surface at 0.0095 separate body contours L0 L6 L20 L10 | L11 L20 L7 L8 L15 L16 L24 L25 L26 L27 L32 L33 L34 L35 L40 L41 L42 L43 L48 L49 L50 L51 L56 L57 L58 L59 L64 L65 L66 L67 L72 L73 L74 L75 L80 L81 L82 L83 L88 L89 L90 L91 L96 L97 L98 L99 L104 L105 L106 L107 L112 L113 L114 L115 L120 L121 L122 L123 L128 L129 L130 L131 L136 L137 L138 L139 L144 L145 L146 L147 L152 L153 L154 L155 L160 L161 L162 L163 L168 L169 L170 L171 L176 L177 L178 L179 L184 L185 L186 L187 L192 L193 L194 L195 L200 L201 L202 L203 L208 L209 L210 L211 L216 L217 L218 L219 L224 L225 L226 L227 L232 L233 L234 L235 L240 L241 L242 L243 L248 L249 L250 L251 L256 L257 L258 L259 L264 L265 L266 L267 L272 L273 L274 L275 L280 L281 L282 L283 L288 L289 L290 L291 L296 L297 L298 L299 L304 L305 L306 L307 L312 L313 L314 L315 L320 L321 L322 L323 L328 L329 L330 L331 L336 L337 L338 L339 L344 L345 L346 L347 L352 L353 L354 L355 L360 L361 L362 L363 L368 L369 L370 L371 L376 L377 L378 L379 L384 L385 L386 L387 L392 L393 L394 L19 L398 L397 L396 L391 L390 L389 L388 L383 L382 L381 L380 L375 L374 L373 L372 L367 L366 L365 L364 L359 L358 L357 L356 L351 L350 L349 L348 L343 L342 L341 L340 L335 L334 L333 L332 L327 L326 L325 L324 L319 L318 L317 L316 L311 L310 L309 L308 L303 L302 L301 L300 L295 L294 L293 L292 L287 L286 L285 L284 L279 L278 L277 L276 L271 L270 L269 L268 L263 L262 L261 L260 L255 L254 L253 L252 L247 L246 L245 L244 L239 L238 L237 L236 L231 L230 L229 L228 L223 L222 L221 L220 L215 L214 L213 L212 L207 L206 L205 L204 L199 L198 L197 L196 L191 L190 L189 L188 L183 L182 L181 L180 L175 L174 L173 L172 L167 L166 L165 L164 L159 L158 L157 L156 L151 L150 L149 L148 L143 L142 L141 L140 L135 L134 L133 L132 L127 L126 L125 L124 L119 L118 L117 L116 L111 L110 L109 L108 L103 L102 L101 L100 L95 L94 L93 L92 L87 L86 L85 L84 L79 L78 L77 L76 L71 L70 L69 L68 L63 L62 L61 L60 L55 L54 L53 L52 L47 L46 L45 L44 L39 L38 L37 L36 L31 L30 L29 L28 L14 L13 L12
sketch "Boceto3" plane through (0, 0, 0) normal (0, 0, 1) x (1, 0, 0)
  line L0 (-0.567, 0.006) -> (-0.917, 0.006) projected
  line L1 (-0.917, 0.006) -> (-0.117, 0.006) construction
  line L2 (0, 0) -> (-0.0078, 0) construction
  line L3 (-1.0262, 0) -> (-1.034, 0) construction
  line L4 (0, 0.006) -> (-1.034, 0.006) construction
  line L5 (0, 0.0136) -> (-1.034, 0.0136)
  line L6 (-1.034, -0.0016) -> (0, -0.0016)
  arc A0 (0, -0.0016) -> (0, 0.0136) centre (0, 0.006) ccw
  arc A1 (-1.034, 0.0136) -> (-1.034, -0.0016) centre (-1.034, 0.006) ccw
  point P0 (-0.517, 0.006)
  point P1 (-0.517, 0)
  point P2 (-0.517, 0.006)
  point P3 (-1.0416, 0.006)
  dimension "d48" = 0.0076
  constraints: 16 end point, 5 point on circle, 4 tangent, 3 parallel, 2 centre point, 2 midpoint, 2 point on line, 1 collinear
  measures "d48" distance of point (-1.042, 0.006) L4.end
extrude "Extrusión10" add sketch "Boceto3" against normal blind 15 separate body
